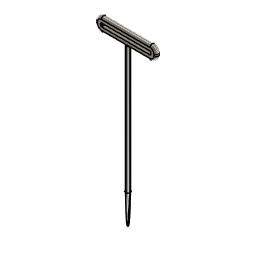
nailEach (Autodesk Fusion 360 design; units mm, degrees)
Autodesk Fusion 360 part; units mm, degrees
sketch "草图1" plane through (0, 0, 0) normal (0, 1, 0) x (1, 0, 0)
  line L0 (0, 0) -> (0, -25.7)
  line L1 (0, -25.7) -> (-4.625, -25.7)
  line L2 (-4.625, -25.7) -> (-4.625, -28)
  line L3 (-4.625, -28) -> (5.375, -28)
  line L4 (5.375, -28) -> (5.375, -25.7)
  line L5 (5.375, -25.7) -> (0.75, -25.7)
  line L6 (0.75, -25.7) -> (0.75, 0)
  line L7 (0.75, 0) -> (0, 0)
  line L8 (0.375, -28) -> (0.375, 0)
  line L9 (0.375, 0) -> (0.375, -0.4348)
  line L10 (0.375, 0) -> (0.75, -5)
  line L11 (0.375, 0) -> (0, -5)
  line L12 (0.75, -5) -> (0, -5)
  dimension "d1" = 2.3
  dimension "d2" = 0.75
  dimension "d3" = 5
  dimension "d4" = 28
  dimension "d5" = 10
  constraint coincident L0.start L7.end
  constraint vertical L0
  constraint perpendicular L0 L1
  constraint perpendicular L1 L2
  constraint perpendicular L2 L3
  constraint perpendicular L2 L5
  constraint perpendicular L1 L6
  constraint perpendicular L0 L7
  constraint perpendicular L4 L5
  constraint midpoint L3 L8.start
  constraint midpoint L7 L8.end
  constraint perpendicular L3 L8
  constraint collinear L1 L5
  constraint coincident L8 L9.end
  constraint coincident L6 L10.end
  constraint coincident L0 L11.end
  constraint perpendicular L6 L12
  measures "d1" distance of L3.end L4.end
  measures "d2" distance of L0 L6
  measures "d3" distance of L7 L10.end
  measures "d4" distance of L3 L8.end
  measures "d5" distance of L2 L4
extrude "拉伸1" add sketch "草图1" along normal blind 0.75 contours L0 L1 L2 L3 L8 L12 | L8 L9 L11 L12 | L8 L9 L10 L12 | L3 L4 L5 L6 L8 L12
fillet "圆角1" radius 1 4 edges at (5.375, 0.375, 28) (5.375, 0.375, 25.7) (-4.625, 0.375, 25.7) (-4.625, 0.375, 28)
fillet "圆角2" radius 0.375 18 edges at (-1.8125, 0, 25.7) (-4.3321, 0, 25.9929) (-4.625, 0, 26.85) (-4.3321, 0, 27.7071) (0.375, 0, 28) (5.0821, 0, 27.7071) (5.375, 0, 26.85) (5.0821, 0, 25.9929) (2.5625, 0, 25.7) (-1.8125, 0.75, 25.7) (-4.3321, 0.75, 25.9929) (-4.625, 0.75, 26.85) (-4.3321, 0.75, 27.7071) (0.375, 0.75, 28) (5.0821, 0.75, 27.7071) (5.375, 0.75, 26.85) (5.0821, 0.75, 25.9929) (2.5625, 0.75, 25.7)
fillet "圆角3" radius 0.325 8 edges at (0.75, 0, 15.5375) (0.75, 0.75, 15.5375) (0, 0.75, 15.5375) (0, 0, 15.5375) (0.5625, 0, 2.5) (0.5625, 0.75, 2.5) (0.1875, 0, 2.5) (0.1875, 0.75, 2.5)
sketch "草图2" plane through (0, 0, 0) normal (0, -1, 0) x (1, 0, 0)
  line L0 (0.425, 26.075) -> (4.375, 26.075)
  arc A0 (4.375, 26.075) -> (5, 26.7) centre (4.375, 26.7) ccw
  line L1 (5, 26.7) -> (5, 27)
  arc A1 (5, 27) -> (4.375, 27.625) centre (4.375, 27) ccw
  line L2 (4.375, 27.625) -> (-3.625, 27.625)
  arc A2 (-3.625, 27.625) -> (-4.25, 27) centre (-3.625, 27) ccw
  line L3 (-4.25, 27) -> (-4.25, 26.7)
  arc A3 (-4.25, 26.7) -> (-3.625, 26.075) centre (-3.625, 26.7) ccw
  line L4 (-3.625, 26.075) -> (0.325, 26.075)
  line L5 (0.325, 26.075) -> (0.325, 5.0122)
  line L6 (0.325, 5.0122) -> (0.375, 4.3455)
  line L7 (0.375, 4.3455) -> (0.425, 5.0122)
  line L8 (0.425, 5.0122) -> (0.425, 26.075)
  line L9 (-3.75, 27) -> (-3.75, 26.7)
  arc A4 (-3.75, 26.7) -> (-3.625, 26.575) centre (-3.625, 26.7) ccw
  line L10 (-3.625, 26.575) -> (-0.075, 26.575)
  line L11 (-0.075, 26.575) -> (0.825, 26.575)
  line L12 (0.825, 26.575) -> (4.375, 26.575)
  arc A5 (4.375, 26.575) -> (4.5, 26.7) centre (4.375, 26.7) ccw
  line L13 (4.5, 26.7) -> (4.5, 27)
  arc A6 (4.5, 27) -> (4.375, 27.125) centre (4.375, 27) ccw
  line L14 (4.375, 27.125) -> (-3.625, 27.125)
  arc A7 (-3.625, 27.125) -> (-3.75, 27) centre (-3.625, 27) ccw
  dimension "d14" = -0.5
extrude "拉伸2" cut sketch "草图2" against normal blind 3 contours L9 A4 L10 L11 L12 A5 L13 A6 L14 A7
equation "d11 = ( 0.75 / 2 ) * 1 mm"
